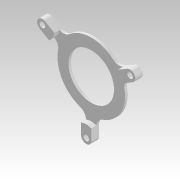
# Autodesk Inventor part: Bracket
Saved by Autodesk Inventor 2020 (Build 240168000, 168)
## iProperties
Created: 2022-01-15
Part Number: Bracket
Material: Generic
Document SubType Name: Modeling
Designer: DDeGo
Density: 1 g/cm^3
Appearance: Default
Author: DDeGo
Autodesk Inventor part; units mm, degrees
ref_plane "YZ Plane" through (0, 0, 0) normal (1, 0, 0) x (0, 1, 0)
ref_plane "XZ Plane" through (0, 0, 0) normal (0, 1, 0) x (-1, 0, 0)
ref_plane "XY Plane" through (0, 0, 0) normal (0, 0, 1) x (1, 0, 0)
sketch "Sketch1" plane through (0, 0, 0) normal (0, 0, 1) x (1, 0, 0)
  circle A0 centre (0, -31) radius 1.6
  circle A1 centre (0, 0) radius 13.5
  circle A2 centre (0, 0) radius 20
  line L0 (0, 0) -> (0, -31) construction
  line L1 (0, -31) -> (0, -7.0396) construction
  line L2 (-3.1, -31) -> (-3.1, -19.7583)
  arc A3 (-3.1, -31) -> (3.1, -31) centre (0, -31) ccw
  line L3 (3.1, -19.7583) -> (3.1, -31)
  circle A4 centre (26.8468, 15.5) radius 1.6
  line L4 (0, 0) -> (26.8468, 15.5) construction
  line L5 (26.8468, 15.5) -> (6.0965, 3.5198) construction
  line L6 (28.3968, 12.8153) -> (18.6612, 7.1945)
  arc A5 (28.3968, 12.8153) -> (25.2968, 18.1847) centre (26.8468, 15.5) ccw
  line L7 (15.5612, 12.5638) -> (25.2968, 18.1847)
  circle A6 centre (-26.8468, 15.5) radius 1.6
  line L8 (0, 0) -> (-26.8468, 15.5) construction
  line L9 (-26.8468, 15.5) -> (-6.0965, 3.5198) construction
  line L10 (-25.2968, 18.1847) -> (-15.5612, 12.5638)
  arc A7 (-25.2968, 18.1847) -> (-28.3968, 12.8153) centre (-26.8468, 15.5) ccw
  line L11 (-18.6612, 7.1945) -> (-28.3968, 12.8153)
  point P0 (18.6612, 7.1945)
  point P1 (15.5612, 12.5638)
  dimension "d4" = 31
  dimension "d5" = 3.2
  dimension "d6" = 27
  dimension "d7" = 40
  dimension "d8" = 1.5
  dimension "d11" = 360
  constraints: 30 end point, 8 centre point, 8 point on circle, 3 point on line, 2 coincident, 2 tangent, 2 vertical, 1 parallel, 40 other
  measures "d4" distance of L0.start L0.end
  measures "d5" diameter of A0
  measures "d6" diameter of A1
  measures "d7" diameter of A2
  measures "d8" radial gap between concentric circles of A0 A3
extrude "Extrusion1" add sketch "Sketch1" along normal blind 1.5
fillet "Fillet1" radius 5 6 edges at (-15.5612, 12.5638, 0.75) (15.5612, 12.5638, 0.75) (18.6612, 7.1945, 0.75) (-18.6612, 7.1945, 0.75) (-3.1, -19.7583, 0.75) (3.1, -19.7583, 0.75)
sketch "Sketch2" plane through (0, 0, 1.5) normal (0, 0, 1) x (1, 0, 0)
  arc A0 (-20.2121, 10.7235) -> (-0.8192, -22.866) centre (-6.2805, -3.626) ccw construction
  arc A1 (0.8192, -22.866) -> (20.2121, 10.7235) centre (6.2805, -3.626) ccw construction
  circle A2 centre (0, 0) radius 13.5 construction
  arc A3 (-20.3166, 10.8312) -> (-0.75, -23.0022) centre (-6.2805, -3.626) ccw
  arc A4 (0.75, -23.0022) -> (19.7139, 11.3928) centre (6.2805, -3.626) ccw
  line L0 (-0.75, -23.0022) -> (0.75, -23.0022)
  line L1 (25.2968, 18.1847) -> (18.9327, 14.5104) projected
  arc A5 (13.1462, 15.0724) -> (18.9327, 14.5104) centre (16.4327, 18.8405) ccw projected
  arc A6 (13.1462, 15.0724) -> (-13.1462, 15.0724) centre (0, 0) ccw projected
  arc A7 (-18.9327, 14.5104) -> (-13.1462, 15.0724) centre (-16.4327, 18.8405) ccw projected
  line L2 (-18.9327, 14.5104) -> (-25.2968, 18.1847) projected
  arc A8 (-25.2968, 18.1847) -> (-28.3968, 12.8153) centre (-26.8468, 15.5) ccw projected
  line L3 (-28.3968, 12.8153) -> (-22.0327, 9.141) projected
  arc A9 (-19.6262, 3.8487) -> (-22.0327, 9.141) centre (-24.5327, 4.8109) ccw projected
  arc A10 (-19.6262, 3.8487) -> (-6.48, -18.9211) centre (0, 0) ccw projected
  arc A11 (-3.1, -23.6514) -> (-6.48, -18.9211) centre (-8.1, -23.6514) ccw projected
  line L4 (-3.1, -23.6514) -> (-3.1, -31) projected
  arc A12 (-3.1, -31) -> (3.1, -31) centre (0, -31) ccw projected
  line L5 (3.1, -31) -> (3.1, -23.6514) projected
  arc A13 (6.48, -18.9211) -> (3.1, -23.6514) centre (8.1, -23.6514) ccw projected
  arc A14 (6.48, -18.9211) -> (19.6262, 3.8487) centre (0, 0) ccw projected
  arc A15 (22.0327, 9.141) -> (19.6262, 3.8487) centre (24.5327, 4.8109) ccw projected
  line L6 (22.0327, 9.141) -> (28.3968, 12.8153) projected
  arc A16 (28.3968, 12.8153) -> (25.2968, 18.1847) centre (26.8468, 15.5) ccw projected
  circle A17 centre (0, -31) radius 1.6 projected
  circle A18 centre (0, 0) radius 13.5 projected
  circle A19 centre (26.8468, 15.5) radius 1.6 projected
  circle A20 centre (-26.8468, 15.5) radius 1.6 projected
  arc A21 (19.5455, 12.1506) -> (-19.7234, 11.3763) centre (0, 7.2521) ccw
  arc A22 (0.7782, -23.0103) -> (20.2955, 10.8516) centre (6.2805, -3.626) ccw
  line L7 (20.2955, 10.8516) -> (19.5455, 12.1506)
  arc A23 (-20.2955, 10.8516) -> (0.0095, -22.7691) centre (-6.2805, -3.626) ccw
  arc A24 (19.5383, 12.1791) -> (-19.5455, 12.1506) centre (0, 7.2521) ccw
  line L8 (-19.5455, 12.1506) -> (-20.2955, 10.8516)
  point P0 (3.1016, -23.5237)
  point P1 (-3.1016, -23.5237)
  point P2 (18.8213, 14.4479)
  point P3 (20.2955, 10.8516)
  point P4 (21.9229, 9.0758)
  point P5 (-21.9229, 9.0758)
  point P6 (-20.3166, 10.8312)
  point P7 (-19.5455, 12.1506)
  point P8 (-18.8213, 14.4479)
  dimension "d16" = 0.15
  dimension "d17" = 0.15
  dimension "d18" = 1.5
  dimension "d21" = 360
  constraints: 12 point on circle, 6 centre point, 6 end point, 1 horizontal, 28 other
  measures "d16" radial gap between concentric circles of A0 A3
  measures "d17" radial gap between concentric circles of A1 A4
  measures "d18" distance of L0.start L0.end
extrude "Extrusion2" add sketch "Sketch2" along normal blind 3 contours A3 A9 L3 A8 L2 A7 A21 L8 A23 | A3 L0 A4 A13 L5 A12 L4 A11 | A5 L1 A16 L6 A15 A4 L7 A21
body "Solid1"
